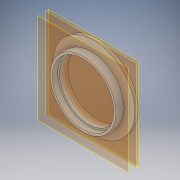
# Autodesk Inventor part: KF50tube_v3
Saved by Autodesk Inventor 2018 (Build 220112000, 112)
## iProperties
Created: 2017-06-29
Part Number: KF50tube_v3
Material: Generic
Document SubType Name: Modeling
Designer: boss
Density: 1 g/cm^3
Appearance: Default
Author: boss
Autodesk Inventor part; units mm, degrees
ref_plane "YZ Plane" through (0, 0, 0) normal (1, 0, 0) x (0, 1, 0)
ref_plane "XZ Plane" through (0, 0, 0) normal (0, 1, 0) x (-1, 0, 0)
sketch "Sketch1" plane through (0, 0, 0) normal (0, 0, 1) x (1, 0, 0)
  circle A0 centre (0, 0) radius 37.465
  dimension "d0" = 74.93
  constraints: 1 centre point, 1 coincident
  measures "d0" diameter of A0
extrude "Extrusion1" add sketch "Sketch1" along normal blind 12.7
sketch "Sketch3" plane through (0, 0, 12.7) normal (0, 0, 1) x (1, 0, 0)
  circle A0 centre (0, 0) radius 26.289
  dimension "d6" = 52.578
  constraints: 1 centre point, 1 coincident
  measures "d6" diameter of A0
extrude "Extrusion3" cut sketch "Sketch3" against normal blind 2.54
sketch "Sketch4" plane through (0, 0, 0) normal (0, 0, -1) x (-1, 0, 0)
  circle A0 centre (0, 0) radius 26.416
  dimension "d9" = 52.832
  constraints: 1 centre point, 1 coincident
  measures "d9" diameter of A0
extrude "Extrusion4" cut sketch "Sketch4" against normal blind 2.54
ref_plane "Work Plane1" through (0, 0, 12.7) normal (0, 0, 1) x (1, 0, 0)
ref_plane "Work Plane3" through (0, 0, 5.2324) normal (0, 0, 1) x (1, 0, 0)
ref_plane "Work Plane5" through (0, 0, 3.048) normal (0, 0, 1) x (1, 0, 0)
sketch "Sketch9" plane through (0, 0, 5.2324) normal (0, 0, 1) x (1, 0, 0)
  circle A0 centre (0, 0) radius 29.845 projected
sketch "Sketch11" plane through (0, 0, 3.048) normal (0, 0, 1) x (1, 0, 0)
  circle A0 centre (0, 0) radius 29.845
  circle A1 centre (0, 0) radius 37.465
  dimension "d42" = 59.69
  dimension "d43" = 74.93
  constraints: 2 centre point, 2 coincident
  measures "d42" diameter of A0
  measures "d43" diameter of A1
extrude "Extrusion7" cut sketch "Sketch11" along normal through all
loft "Loft5" add profiles "Sketch9" section 2 edges at (-37.465, 0, 3.048)
sketch "Sketch12" plane through (0, 0, 12.7) normal (0, 0, 1) x (1, 0, 0)
  circle A0 centre (0, 0) radius 27.94
  circle A1 centre (0, 0) radius 26.289
  dimension "d50" = 55.88
  constraints: 2 centre point, 2 coincident
  measures "d50" diameter of A0
extrude "Extrusion8" cut sketch "Sketch12" against normal blind 5.08
sketch "Sketch2" plane through (0, 0, 12.7) normal (0, 0, 1) x (1, 0, 0)
  circle A0 centre (0, 0) radius 26.416
  dimension "d3" = 52.832
  constraints: 1 centre point, 1 coincident
  measures "d3" diameter of A0
extrude "Extrusion2" cut sketch "Sketch2" against normal blind 50.8
body "Solid1"
